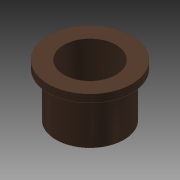
# Autodesk Inventor part: Flange_Sleeve_Bearing_5448T5
Saved by Autodesk Inventor 2015 (Build 190159000, 159)
## iProperties
Created: 2015-01-04
Part Number: Flange_Sleeve_Bearing_5448T5
Material: Bronze, Cast
Document SubType Name: Modeling
Designer: Drew
Density: 8.87 g/cm^3
Appearance: Bronze - Satin
Author: Drew
Autodesk Inventor part; units mm, degrees
ref_plane "YZ Plane" through (0, 0, 0) normal (1, 0, 0) x (0, 1, 0)
ref_plane "XZ Plane" through (0, 0, 0) normal (0, 1, 0) x (-1, 0, 0)
ref_plane "XY Plane" through (0, 0, 0) normal (0, 0, 1) x (1, 0, 0)
sketch "Sketch1" plane through (0, 0, 0) normal (1, 0, 0) x (0, 1, 0)
  line L0 (0, -5) -> (0, -8)
  line L1 (0, -8) -> (-1.5, -8)
  line L2 (-1.5, -8) -> (-1.5, -6.5)
  line L3 (-1.5, -6.5) -> (-10, -6.5)
  line L4 (-10, -6.5) -> (-10, -5)
  line L5 (-10, -5) -> (0, -5)
  line L6 (0, 5.637) -> (0, -6.8088)
  line L7 (5.7696, 0) -> (-13.4996, 0)
  point P0 (0, 0)
  point P1 (0, -0.5859)
  dimension "d0" = 5
  dimension "d2" = 1.5
  dimension "d3" = 10
  dimension "d4" = 1.5
  dimension "d5" = 8
  constraints: 16 end point, 5 perpendicular, 2 point on line, 2 vertical, 1 horizontal, 1 midpoint
  measures "d0" distance from line of point (0, 0) L5
  measures "d2" distance of L0.end L1.end
  measures "d3" distance between parallel lines of L0 L4
  measures "d4" distance between parallel lines of L3 L5
  measures "d5" distance from line of point (0, 0) L1
revolve "Revolution1" add sketch "Sketch1" angle 360 about axis through (0, 5.7696, 0) along (0, -1, 0)
equation "\"d2\" = d4"
body "Solid1"
